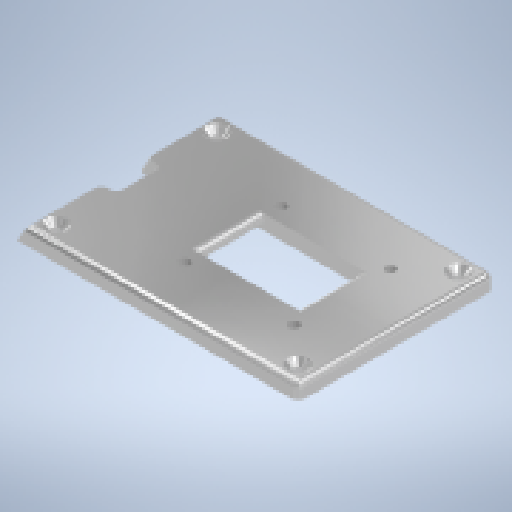
# Autodesk Inventor part: SchlittenDeckel
Saved by Autodesk Inventor 2025 (Build 290162010, 162A)
## iProperties
Created: 2024-11-26
Part Number: SchlittenDeckel
Material: Aluminium 6061(1)
Document SubType Name: Modeling
Designer: Admin
Density: 2.7 g/cm^3
Appearance: Aluminium - flach(1)
Author: Admin
Autodesk Inventor part; units mm, degrees
ref_plane "YZ Plane" through (0, 0, 0) normal (1, 0, 0) x (0, 1, 0)
ref_plane "XZ Plane" through (0, 0, 0) normal (0, 1, 0) x (-1, 0, 0)
ref_plane "XY Plane" through (0, 0, 0) normal (0, 0, 1) x (1, 0, 0)
sketch "Skizze1" plane through (0, 0, 0) normal (0, 0, 1) x (1, 0, 0)
  line L0 (300, -63) -> (210, -63)
  line L1 (210, -63) -> (210, -38)
  line L2 (210, -38) -> (215, -38)
  line L3 (215, -38) -> (215, -23)
  line L4 (215, -23) -> (210, -23)
  line L5 (210, -23) -> (210, 2)
  line L6 (210, 2) -> (300, 2)
  line L7 (300, -63) -> (300, 2)
  dimension "d59" = 90
  dimension "d60" = 25
  dimension "d61" = 5
  dimension "d62" = 15
  constraints: 16 end point, 6 perpendicular, 2 point on line, 1 collinear, 1 horizontal, 1 other
  measures "d59" distance of L0.start L0.end
  measures "d60" distance of L0.end L1.end
  measures "d61" distance of L1.end L2.end
  measures "d62" distance of L2.end L3.end
extrude "Extrusion1" add sketch "Skizze1" along normal blind 5
sketch "Skizze3" plane through (0, 0, 5) normal (0, 0, 1) x (1, 0, 0)
  line L0 (282, -14.5) -> (246, -14.5)
  line L1 (246, -14.5) -> (246, -46.5)
  line L2 (246, -46.5) -> (282, -46.5)
  line L3 (282, -46.5) -> (282, -14.5)
  line L4 (282, -30.5) -> (300, -30.5)
  line L5 (300, -63) -> (300, 2) projected
  point P0 (0, 0)
  dimension "d15" = 36
  dimension "d16" = 32
  dimension "d17" = 18
  constraints: 10 end point, 4 coincident, 2 midpoint, 2 parallel, 2 perpendicular, 1 horizontal
  measures "d15" distance of L2.end L1.end
  measures "d16" distance of L1.end L0.end
  measures "d17" distance of L4.end L4.start
hole "hebel" at (282, -46.5, 5) at (282, -14.5, 5) at (246, -14.5, 5) at (246, -46.5, 5) direction (0, 0, -1) diameter 3.242 end through all
fillet "Rundung2" radius 2 4 edges at (215, -23, 2.5) (215, -38, 2.5) (210, -38, 2.5) (210, -23, 2.5)
fillet "Rundung3" radius 2 5 edges at (255, 2, 5) (300, -30.5, 5) (255, -63, 5) (300, 2, 2.5) (300, -63, 2.5)
sketch "Skizze10" plane through (210, 2, 0) normal (0, 1, 0) x (1, 0, 0)
  line L0 (88, 0) -> (0, 0) construction
  line L1 (0, -5) -> (88, -5) construction
  line L2 (0, 0) -> (2.8868, -5)
  line L3 (0, 0) -> (5.7735, 0) construction
  point P0 (-210, 0)
  dimension "d79" = 60
  constraints: 4 end point, 1 equal length, 1 horizontal, 1 point on line
  measures "d79" angle of L2 L3
sketch "Skizze11" plane through (0, 0, 0) normal (0, 0, -1) x (-1, 0, 0)
  line L0 (-207.1132, 2) -> (-207.1132, -21)
  arc A0 (-209.1132, -23) -> (-207.1132, -21) centre (-209.1132, -21) ccw
  line L1 (-212.1132, -25) -> (-212.1132, -36)
  arc A1 (-210.1132, -23) -> (-212.1132, -25) centre (-210.1132, -25) ccw
  line L2 (-209.1132, -23) -> (-210.1132, -23)
  arc A2 (-212.1132, -36) -> (-210.1132, -38) centre (-210.1132, -36) ccw
  line L3 (-210.1132, -38) -> (-209.1132, -38)
  arc A3 (-207.1132, -40) -> (-209.1132, -38) centre (-209.1132, -40) ccw
  line L4 (-207.1132, -40) -> (-207.1132, -63)
  line L5 (-210, 2) -> (-210, -21) projected
  arc A4 (-212, -23) -> (-210, -21) centre (-212, -21) ccw projected
  line L6 (-212, -23) -> (-213, -23) projected
  arc A5 (-213, -23) -> (-215, -25) centre (-213, -25) ccw projected
  line L7 (-215, -25) -> (-215, -36) projected
  line L8 (-213, -38) -> (-212, -38) projected
  arc A6 (-215, -36) -> (-213, -38) centre (-213, -36) ccw projected
  arc A7 (-210, -40) -> (-212, -38) centre (-212, -40) ccw projected
  line L9 (-210, -40) -> (-210, -63) projected
  line L10 (-298, 2) -> (-210, 2) projected
  line L11 (-210, 2) -> (-207.1132, 2)
  line L12 (-210, -63) -> (-207.1132, -63)
  line L13 (-210, 2) -> (-212.8868, 2) projected
  point P0 (0, 0)
  constraints: 14 end point, 8 point on circle, 7 equal length, 7 tangent, 4 centre point, 4 parallel, 2 collinear, 2 equal radius, 1 perpendicular
sweep "Sweeping2" add profiles "Skizze11" path "Skizze10"
sketch "Skizze8" plane through (0, 0, 5) normal (0, 0, 1) x (1, 0, 0)
  line L0 (294, -4) -> (294, -30.5) construction
  line L1 (294, -30.5) -> (294, -57) construction
  line L2 (298, 0) -> (298, -61) construction
  line L3 (298, -30.5) -> (294, -30.5) construction
  line L4 (294, -4) -> (294, 0) construction
  line L5 (210, 0) -> (298, 0) construction
  line L6 (214, -4) -> (214, 0)
  line L7 (214, -57) -> (214, -30.5)
  line L8 (214, -30.5) -> (214, -4)
  line L9 (214, -4) -> (210, -4)
  line L10 (210, 0) -> (210, -21) projected
  point P0 (0, 0)
  dimension "d15" = 36
  dimension "d16" = 32
  dimension "d17" = 18
  dimension "d65" = 4
  constraints: 16 end point, 5 equal length, 4 point on line, 2 collinear, 2 perpendicular, 2 vertical, 1 horizontal, 1 midpoint
  measures "d65" distance of L3.start L0.end
hole "Bohrung5" at (294, -4, 5) at (294, -57, 5) at (214, -4, 5) at (214, -57, 5) direction (0, 0, -1) diameter 3.2 end through all countersink diameter 7 countersink angle 90
fillet "Rundung5" radius 2 2 edges at (211.4434, -63, 5) (211.4434, 2, 5)
sketch "Skizze12" plane through (0, 0, 5) normal (0, 0, 1) x (1, 0, 0)
  circle A0 centre (282, -14.5) radius 1.621 construction
  circle A1 centre (246, -14.5) radius 1.621 construction
  circle A2 centre (282, -46.5) radius 1.621 construction
  circle A3 centre (246, -46.5) radius 1.621 construction
  line L0 (282, -14.5) -> (246, -46.5) construction
  line L1 (246, -46.5) -> (246, -14.5) construction
  line L2 (246, -14.5) -> (282, -46.5) construction
  line L3 (249, -20.5) -> (275.82, -20.5) construction
  line L4 (275.82, -20.5) -> (275.82, -40.5) construction
  line L5 (275.82, -40.5) -> (249, -40.5) construction
  line L6 (249, -40.5) -> (249, -20.5) construction
  line L7 (264, -30.5) -> (249, -30.5) construction
  line L8 (264, -30.5) -> (275.82, -30.5) construction
  line L9 (248, -19.5) -> (276.82, -19.5)
  line L10 (276.82, -19.5) -> (276.82, -41.5)
  line L11 (276.82, -41.5) -> (248, -41.5)
  line L12 (248, -41.5) -> (248, -19.5)
  line L13 (249, -30.5) -> (248, -30.5) construction
  line L14 (262.41, -19.5) -> (262.41, -20.5) construction
  line L15 (262.41, -40.5) -> (262.41, -41.5) construction
  line L16 (275.82, -30.5) -> (276.82, -30.5) construction
  point P0 (0, 0)
  dimension "d83" = 20
  dimension "d85" = 11.82
  dimension "d86" = 15
  dimension "d87" = 1
  constraints: 34 end point, 9 midpoint, 6 perpendicular, 4 parallel, 3 equal length, 2 horizontal, 1 point on line, 1 vertical
  measures "d83" distance of L3.end L4.end
  measures "d85" distance of L7.start L8.end
  measures "d86" distance of L7.start L7.end
  measures "d87" distance between parallel lines of L12 L6
sketch "Skizze14" plane through (0, 0, 0) normal (0, 0, -1) x (-1, 0, 0)
  circle A0 centre (-246, -14.5) radius 1.621 construction
  circle A1 centre (-282, -14.5) radius 1.621 construction
  circle A2 centre (-246, -46.5) radius 1.621 construction
  circle A3 centre (-282, -46.5) radius 1.621 construction
  line L0 (-246, -14.5) -> (-282, -46.5) construction
  line L1 (-282, -14.5) -> (-246, -46.5) construction
  line L2 (-246, -46.5) -> (-246, -14.5) construction
  line L3 (-249, -30.5) -> (-248, -30.5) construction
  line L4 (-243, -19.5) -> (-278.64, -19.5)
  line L5 (-278.64, -19.5) -> (-278.64, -41.5)
  line L6 (-278.64, -41.5) -> (-243, -41.5)
  line L7 (-243, -41.5) -> (-243, -19.5)
  line L8 (-244, -20.5) -> (-277.64, -20.5) construction
  line L9 (-277.64, -20.5) -> (-277.64, -40.5) construction
  line L10 (-277.64, -40.5) -> (-244, -40.5) construction
  line L11 (-244, -40.5) -> (-244, -20.5) construction
  line L12 (-275.82, -40.5) -> (-249, -40.5) construction
  line L13 (-249, -20.5) -> (-275.82, -20.5) construction
  line L14 (-277.64, -30.5) -> (-278.64, -30.5) construction
  line L15 (-244, -30.5) -> (-243, -30.5) construction
  line L16 (-260.82, -19.5) -> (-260.82, -20.5) construction
  point P0 (0, 0)
  point P1 (-264, -30.5)
  point P2 (-264, -30.5)
  dimension "d88" = 20
  dimension "d89" = 13.64
  constraints: 22 end point, 7 midpoint, 4 parallel, 4 perpendicular, 3 equal length, 2 collinear, 2 horizontal, 1 point on line
  measures "d88" distance from line of L11 point (-264, -30.5)
  measures "d89" distance from line of L9 point (-264, -30.5)
loft "Erhebung1" cut profiles "Skizze12", "Skizze14"
fillet "Rundung6" radius 2 2 edges at (248, -30.5, 5) (276.82, -30.5, 5)
